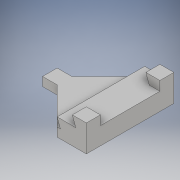
# Autodesk Inventor part: Tirador
Saved by Autodesk Inventor 2017 (Build 210142000, 142)
## iProperties
Created: 2017-01-19
Part Number: Tirador
Material: Generic
Document SubType Name: Modeling
Designer: A. Matías Quezada
Density: 1 g/cm^3
Appearance: Default
Author: A. Matías Quezada
Autodesk Inventor part; units mm, degrees
ref_plane "YZ Plane" through (0, 0, 0) normal (1, 0, 0) x (0, 1, 0)
ref_plane "XZ Plane" through (0, 0, 0) normal (0, 1, 0) x (-1, 0, 0)
ref_plane "XY Plane" through (0, 0, 0) normal (0, 0, 1) x (1, 0, 0)
sketch "Sketch1" plane through (0, 0, 0) normal (0, 0, 1) x (1, 0, 0)
  line L0 (0, 0) -> (-10, 0)
  line L1 (-10, 0) -> (-10, 30)
  line L2 (-10, 30) -> (0, 30)
  line L3 (0, 30) -> (0, 0)
  line L4 (-10, 30) -> (-22.5, 17.5)
  line L5 (-22.5, 17.5) -> (-27.5, 17.5)
  line L6 (-27.5, 17.5) -> (-27.5, 12.5)
  line L7 (-27.5, 12.5) -> (-22.5, 12.5)
  line L8 (-22.5, 12.5) -> (-10, 0)
  dimension "d0" = 10
  dimension "d1" = 30
  dimension "d2" = 5
  dimension "d3" = 45
  constraints: 18 end point, 3 equal length, 3 perpendicular, 2 horizontal, 2 parallel
  measures "d0" distance of L1.end L2.end
  measures "d1" distance of L0.end L1.end
  measures "d2" distance of L5.end L6.end
  measures "d3" angle of L1 L8
extrude "Gancho" add sketch "Sketch1" along normal blind 3
sketch "Sketch2" plane through (0, 0, 3) normal (0, 0, 1) x (1, 0, 0)
  line L0 (-10, 0) -> (0, 0) projected
  line L1 (0, 0) -> (0, 30) projected
  line L2 (0, 30) -> (-10, 30) projected
  line L3 (-10, 30) -> (-10, 0)
  constraints: 2 end point, 1 vertical
extrude "Deslizador" add sketch "Sketch2" along normal blind 3
draft "Agarre Deslizador" angle -20 pull direction (0, 0, 1) faces at (-10, 10, 5) fixed edges at (-10, 15, 6)
sketch "Sketch3" plane through (0, 0, 6) normal (0, 0, 1) x (1, 0, 0)
  line L0 (0, 30) -> (-10, 30) projected
  line L1 (-4.8, 30) -> (-4.8, 25.2)
  line L2 (-4.8, 25.2) -> (0, 25.2)
  line L3 (0, 4.8) -> (-4.8, 4.8)
  line L4 (-4.8, 4.8) -> (-4.8, 0)
  line L5 (-10, 0) -> (0, 0) projected
  line L6 (0, 0) -> (0, 30) projected
  dimension "d9" = 4.8
  constraints: 8 end point, 4 point on line, 3 equal length, 3 perpendicular, 1 horizontal
  measures "d9" distance of L1.start L1.end
extrude "Hoja" add sketch "Sketch3" along normal blind 3.2
draft "Agarre Hoja 1" angle -20 pull direction (0, 0, 1) faces at (-4.8, 28.4, 7.0667) fixed edges at (-4.8, 27.6, 9.2)
draft "Agarre Hoja 2" angle -20 pull direction (0, 0, 1) faces at (-4.8, 3.2, 7.0667) fixed edges at (-4.8, 2.4, 9.2)
equation "\"d0\" = tirador_deslizador_largo"
equation "\"d1\" = tirador_ancho"
equation "\"d2\" = tirador_gancho_ancho"
equation "\"d3\" = tirador_gancho_angulo"
equation "\"d4\" = tirador_gancho_grosor"
equation "\"d6\" = tirador_deslizador_grosor"
equation "\"d8\" = tirador_deslizador_agarre"
equation "\"d9\" = tirador_diente_ancho"
equation "\"d10\" = tirador_diente_grosor"
equation "\"d12\" = tirador_diente_agarre"
equation "\"d13\" = tirador_diente_agarre"
equation "\"tirador_deslizador_largo\" = 10"
equation "\"tirador_ancho\" = 30"
equation "\"tirador_gancho_ancho\" = 5"
equation "\"tirador_gancho_angulo\" = 45deg"
equation "\"tirador_gancho_grosor\" = 3"
equation "\"tirador_deslizador_grosor\" = 3"
equation "\"tirador_deslizador_agarre\" = -20deg"
equation "\"tirador_diente_ancho\" = 4.8"
equation "\"tirador_diente_grosor\" = 3.2"
equation "\"tirador_diente_agarre\" = -20deg"
body "Solid1"
